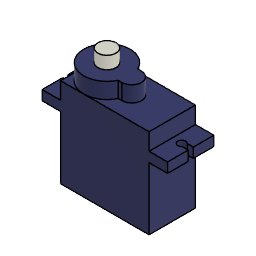
Servo Motor SG90 (Autodesk Fusion 360 design; units mm, degrees)
Autodesk Fusion 360 part; units mm, degrees
sketch "Sketch1" plane through (0, 0, 0) normal (0, 0, 1) x (1, 0, 0)
  circle A0 centre (0, 0) radius 2.3
  circle A1 centre (0, 0) radius 5.9
  line L0 (5.9, 5.9) -> (-5.9, 5.9) construction
  line L1 (-5.9, 5.9) -> (-5.9, -5.9) construction
  line L2 (-5.9, -5.9) -> (5.9, -5.9) construction
  line L3 (5.9, -5.9) -> (5.9, 5.9) construction
  line L4 (5.9, 5.9) -> (-5.9, -5.9) construction
  line L5 (-5.9, 5.9) -> (5.9, -5.9) construction
  line L6 (-5.9, 5.9) -> (16.6, 5.9)
  line L7 (16.6, 5.9) -> (16.6, -5.9)
  line L8 (16.6, -5.9) -> (-5.9, -5.9)
  line L9 (-5.9, -5.9) -> (-5.9, 5.9)
  circle A2 centre (6.3, 0) radius 2.5
  line L10 (6.3, 2.5) -> (5.3442, 2.5)
  line L11 (6.3, -2.5) -> (5.3442, -2.5)
  line L12 (5.35, 7) -> (5.35, -7) construction
  line L13 (-5.9, 5.9) -> (-10.6, 5.9)
  line L14 (-10.6, 5.9) -> (-10.6, 0.65)
  line L15 (-10.6, 0.65) -> (-8.3, 0.65)
  line L16 (-8.3, 0.65) -> (-8.3, -0.65)
  line L17 (-8.3, -0.65) -> (-10.6, -0.65)
  line L18 (-10.6, -0.65) -> (-10.6, -5.9)
  line L19 (-10.6, -5.9) -> (-5.9, -5.9)
  circle A3 centre (-8.3, 0) radius 1
  line L20 (16.6, 5.9) -> (21.3, 5.9)
  line L21 (21.3, 5.9) -> (21.3, 0.65)
  line L22 (21.3, 0.65) -> (19, 0.65)
  circle A4 centre (19, 0) radius 1
  line L23 (19, -0.65) -> (21.3, -0.65)
  line L24 (21.3, -0.65) -> (21.3, -5.9)
  line L25 (21.3, -5.9) -> (16.6, -5.9)
  dimension "d1" = 4.6
  dimension "d2" = 11.8
  dimension "d3" = 11.8
  dimension "d4" = 11.8
  dimension "d5" = 22.5
  dimension "d6" = 11.8
  dimension "d7" = 5
  dimension "d8" = 10.3
  dimension "d9" = 11.25
  dimension "d10" = 4.7
  dimension "d11" = 5.25
  dimension "d12" = 2.3
  dimension "d13" = 1.3
  dimension "d14" = 2
  constraint coincident A0.centre A1.centre
  constraint concentric A0 A1
  constraint horizontal L0
  constraint perpendicular L0 L1
  constraint parallel L0 L2
  constraint parallel L1 L3
  constraint coincident L4 A0.centre
  constraint coincident L5 A0.centre
  constraint horizontal L6
  constraint vertical L7
  constraint horizontal L8
  constraint vertical L9
  constraint coincident A2 L10.start
  constraint coincident A1 L10.end
  constraint perpendicular L3 L10
  constraint coincident A2 L11.start
  constraint coincident A1 L11.end
  constraint tangent A2 L11
  constraint perpendicular L3 L11
  constraint perpendicular L8 L12
  constraint perpendicular L9 L13
  constraint perpendicular L13 L14
  constraint perpendicular L14 L15
  constraint perpendicular L15 L16
  constraint perpendicular L16 L17
  constraint perpendicular L2 L18
  constraint perpendicular L9 L19
  constraint midpoint L16 A3.centre
  constraint symmetric L0.end L12 L6.end
  constraint symmetric L1.end L12 L7.end
  constraint symmetric L12 L13.end L20.end
  constraint symmetric L12 L14.end L21.end
  constraint symmetric L12 L15.end L22.end
  constraint symmetric L12 L16.end L23.start
  constraint symmetric L12 L17.end L23.end
  constraint symmetric L12 L18.end L24.end
  constraint symmetric L12 A3 A4
  measures "d1" diameter of A0
  measures "d2" diameter of A1
  measures "d3" distance of L1.end L2.end
  measures "d4" distance of L0.end L1.end
  measures "d5" distance of L0.end L6.end
  measures "d6" distance of L0.end L1.end
  measures "d7" diameter of A2
  measures "d8" distance of L7 A2.centre
  measures "d9" distance of L7 L12
  measures "d10" distance of L0.end L13.end
  measures "d11" distance of L13.end L14.end
  measures "d12" distance of L14.end L15.end
  measures "d13" distance of L15.end L16.end
  measures "d14" diameter of A3
extrude "Extrude1" add sketch "Sketch1" along normal blind 22.7 contours A0 | A1 A2 | A1 A2 | A1 A2 | A1 A2 L10 | A1 A2 L11 | A1 L6 L7 L8 A2 L10 L11 | A1 L6 L9 | A1 L8 L9 makes body 1 in component "Housing"
extrude "Extrude2" add sketch "Sketch1" along normal blind 4 from surface at 22.7 contours A1 A2 | A1 A2 | A1 A2 | A1 A2 L10 | A1 A2 L11 bodies 1 in component "Housing"
extrude "Extrude3" add sketch "Sketch1" along normal blind 2.5 from surface at 15.9 contours L9 L13 L14 L15 L17 L18 L19 A3 | L7 L20 L21 L22 A4 L23 L24 L25 bodies 1 in component "Housing"
extrude "Extrude1'" add sketch "Sketch1" along normal blind 7.2 from surface at 22.7 separate body contours A0 makes body 2 in component "Shaft"
sketch "Sketch2" plane through (-5.9, 0, 0) normal (-1, 0, 0) x (0, -1, 0)
  line L0 (5.9, 15.9) -> (-5.9, 15.9)
  line L1 (-5.9, 15.9) -> (-5.9, 0)
  line L2 (-5.9, 0) -> (5.9, 0)
  line L3 (5.9, 0) -> (5.9, 15.9)
  line L4 (0, 0) -> (-1.75, 0) construction
  line L5 (-1.75, 0) -> (1.75, 0)
  line L6 (1.75, 0) -> (1.75, 4.5)
  line L7 (1.75, 4.5) -> (-1.75, 4.5)
  line L8 (-1.75, 4.5) -> (-1.75, 0)
  dimension "d26" = 1.75
  dimension "d27" = 3.5
  dimension "d28" = 4.5
  constraint coincident L4.start origin
  constraint parallel L2 L4
  constraint horizontal L5
  constraint vertical L6
  constraint horizontal L7
  constraint vertical L8
  measures "d26" distance of L4.start L4.end
  measures "d27" distance of L4.end L5.end
  measures "d28" distance of L4.end L7.end
extrude "Extrude4" cut sketch "Sketch2" against normal blind 1.5 contours L2 L5 L6 L7 L8 bodies 1 in component "Housing"
component "Housing" placed x (1, 0, 0) y (0, 1, 0) z (0, 0, 1) at (0, 0, 0)
component "Shaft" placed x (1, 0, 0) y (0, -1, 0) z (0, 0, -1) at (0, 0, 52.6)
equation "d26 = ( 3.5 / 2 ) * 1 mm"
